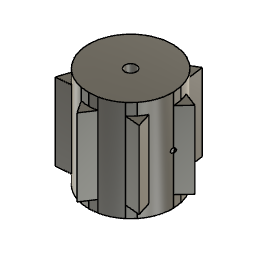
engranaje v5 (Autodesk Fusion 360 design; units mm, degrees)
Autodesk Fusion 360 part; units mm, degrees
sketch "Sketch1" plane through (0, 0, 0) normal (0, 0, 1) x (1, 0, 0)
  circle A0 centre (0, 0) radius 25
  line L0 (0, 25) -> (4.9749, 24.5)
  line L1 (0, 25) -> (-4.9749, 24.5)
  line L2 (0, -25) -> (0, -32)
  line L3 (0, -25) -> (-4.9749, -24.5)
  line L4 (0, -25) -> (0, -32)
  line L5 (0, -32) -> (-4.9749, -24.5)
  line L6 (0, -25) -> (4.9749, -24.5)
  line L7 (0, -32) -> (4.9749, -24.5)
  line L8 (25.0186, -19.9517) -> (16.053, -19.1651)
  line L9 (19.5458, -15.5872) -> (25.0186, -19.9517)
  line L10 (19.5458, -15.5872) -> (16.053, -19.1651)
  circle A1 centre (0, 0) radius 25
  line L11 (25.0186, -19.9517) -> (22.2567, -11.3859)
  line L12 (31.1977, 7.1207) -> (24.9928, 0.6016)
  line L13 (24.3732, 5.563) -> (31.1977, 7.1207)
  line L14 (24.3732, 5.563) -> (24.9928, 0.6016)
  circle A2 centre (0, 0) radius 25
  line L15 (31.1977, 7.1207) -> (22.7787, 10.302)
  line L16 (13.8843, 28.831) -> (15.1124, 19.9152)
  line L17 (10.8471, 22.5242) -> (13.8843, 28.831)
  line L18 (10.8471, 22.5242) -> (15.1124, 19.9152)
  circle A3 centre (0, 0) radius 25
  line L19 (13.8843, 28.831) -> (6.1479, 24.2323)
  line L20 (-13.8843, 28.831) -> (-6.1479, 24.2323)
  line L21 (-10.8471, 22.5242) -> (-13.8843, 28.831)
  line L22 (-10.8471, 22.5242) -> (-6.1479, 24.2323)
  circle A4 centre (0, 0) radius 25
  line L23 (-13.8843, 28.831) -> (-15.1124, 19.9152)
  line L24 (-31.1977, 7.1207) -> (-22.7787, 10.302)
  line L25 (-24.3732, 5.563) -> (-31.1977, 7.1207)
  line L26 (-24.3732, 5.563) -> (-22.7787, 10.302)
  circle A5 centre (0, 0) radius 25
  line L27 (-31.1977, 7.1207) -> (-24.9928, 0.6016)
  line L28 (-25.0186, -19.9517) -> (-22.2567, -11.3859)
  line L29 (-19.5458, -15.5872) -> (-25.0186, -19.9517)
  line L30 (-19.5458, -15.5872) -> (-22.2567, -11.3859)
  circle A6 centre (0, 0) radius 25
  line L31 (-25.0186, -19.9517) -> (-16.053, -19.1651)
  dimension "d1" = 50
  dimension "d2" = 5
  dimension "d3" = 7
  dimension "d4" = 5
  dimension "d5" = 5
  dimension "d7" = 360
  constraint coincident A0.centre A1.centre
  constraint coincident A0 L0.start
  constraint coincident A0 L0.end
  constraint coincident A0 L1.end
  constraint coincident A0 L2.start
  constraint vertical L2
  constraint coincident A0 L3.end
  constraint coincident A0 L6.end
  measures "d1" diameter of A0
  measures "d2" distance of L0.start L0.end
  measures "d3" distance of L2.start L2.end
  measures "d4" distance of L2.start L3.end
  measures "d5" distance of L2.start L6.end
extrude "Extrude1" add sketch "Sketch1" along normal blind 60 contours A0 L0 L1 L3 L6 L10 A1 L14 A2 L18 A3 L22 A4 L26 A5 L30 A6 | A0 A1 L12 L13 A2 A3 A4 A5 A6 | A0 L9 A1 L11 A2 A3 A4 A5 A6 | A0 A1 L13 A2 L15 A3 A4 A5 A6 | A0 L8 L9 A1 A2 A3 A4 A5 A6 | A0 A1 A2 L16 L17 A3 A4 A5 A6 | A0 L2 L4 L7 A1 A2 A3 A4 A5 A6 | A0 A1 A2 L17 A3 L19 A4 A5 A6 | A0 L2 L4 L5 A1 A2 A3 A4 A5 A6 | A0 A1 A2 A3 A4 A5 L29 A6 L31 | A0 A1 A2 A3 A4 A5 L28 L29 A6 | A0 A1 A2 A3 L20 L21 A4 A5 A6 | A0 A1 A2 A3 A4 L25 A5 L27 A6 | A0 A1 A2 A3 L21 A4 L23 A5 A6 | A0 A1 A2 A3 A4 L24 L25 A5 A6
sketch "Sketch2" plane through (0, 0, 60) normal (0, 0, 1) x (-1, 0, 0)
  arc A0 (6.1479, -24.2323) -> (10.8471, -22.5242) centre (0, 0) ccw
  line L0 (6.1479, -24.2323) -> (13.8843, -28.831)
  line L1 (13.8843, -28.831) -> (15.1124, -19.9152)
  arc A1 (15.1124, -19.9152) -> (22.7787, -10.302) centre (0, 0) ccw
  line L2 (22.7787, -10.302) -> (24.3732, -5.563)
  arc A2 (22.7787, -10.302) -> (24.3732, -5.563) centre (0, 0) ccw
  line L3 (22.7787, -10.302) -> (31.1977, -7.1207)
  line L4 (31.1977, -7.1207) -> (24.9928, -0.6016)
  arc A3 (24.9928, -0.6016) -> (22.2567, 11.3859) centre (0, 0) ccw
  line L5 (22.2567, 11.3859) -> (19.5458, 15.5872)
  arc A4 (22.2567, 11.3859) -> (19.5458, 15.5872) centre (0, 0) ccw
  line L6 (22.2567, 11.3859) -> (25.0186, 19.9517)
  line L7 (25.0186, 19.9517) -> (16.053, 19.1651)
  arc A5 (16.053, 19.1651) -> (4.9749, 24.5) centre (0, 0) ccw
  line L8 (4.9749, 24.5) -> (0, 25)
  line L9 (0, 25) -> (-4.9749, 24.5)
  arc A6 (-4.9749, 24.5) -> (-16.053, 19.1651) centre (0, 0) ccw
  line L10 (-16.053, 19.1651) -> (-19.5458, 15.5872)
  arc A7 (-16.053, 19.1651) -> (-19.5458, 15.5872) centre (0, 0) ccw
  line L11 (-16.053, 19.1651) -> (-25.0186, 19.9517)
  line L12 (-25.0186, 19.9517) -> (-22.2567, 11.3859)
  arc A8 (-22.2567, 11.3859) -> (-24.9928, -0.6016) centre (0, 0) ccw
  line L13 (-24.9928, -0.6016) -> (-24.3732, -5.563)
  arc A9 (-24.9928, -0.6016) -> (-24.3732, -5.563) centre (0, 0) ccw
  line L14 (-24.9928, -0.6016) -> (-31.1977, -7.1207)
  line L15 (-31.1977, -7.1207) -> (-22.7787, -10.302)
  arc A10 (-22.7787, -10.302) -> (-15.1124, -19.9152) centre (0, 0) ccw
  line L16 (-15.1124, -19.9152) -> (-10.8471, -22.5242)
  arc A11 (-15.1124, -19.9152) -> (-10.8471, -22.5242) centre (0, 0) ccw
  line L17 (-15.1124, -19.9152) -> (-13.8843, -28.831)
  line L18 (-13.8843, -28.831) -> (-6.1479, -24.2323)
  arc A12 (-6.1479, -24.2323) -> (-4.9749, -24.5) centre (0, 0) ccw
  line L19 (-4.9749, -24.5) -> (0, -25)
  line L20 (0, -25) -> (4.9749, -24.5)
  arc A13 (4.9749, -24.5) -> (6.1479, -24.2323) centre (0, 0) ccw
  line L21 (6.1479, -24.2323) -> (10.8471, -22.5242)
  circle A14 centre (0, 0) radius 32
  circle A15 centre (0, 0) radius 25
  constraint concentric A0 A14
  constraint coincident L14.end A14
  constraint concentric A0 A15
  constraint coincident L13.end A15
extrude "Extrude2" cut sketch "Sketch2" against normal blind 7 contours A0 L0 L1 A15 | L0 L18 A12 A13 A14 A15 | L1 A1 L3 A14 A15 | L15 A10 L17 A14 A15 | A11 L17 L18 A15 | A2 L3 L4 A15 | L4 A3 L6 A14 A15 | L12 A8 L14 A14 A15 | A9 L14 L15 A15 | L7 A5 A6 L11 A14 A15 | A7 L11 L12 A15 | A4 L6 L7 A15
sketch "Sketch3" plane through (0, 0, 0) normal (0, 0, -1) x (1, 0, 0)
  arc A0 (-10.8471, -22.5242) -> (-6.1479, -24.2323) centre (0, 0) ccw
  line L0 (-10.8471, -22.5242) -> (-6.1479, -24.2323)
  arc A1 (-6.1479, -24.2323) -> (-4.9749, -24.5) centre (0, 0) ccw
  line L1 (-4.9749, -24.5) -> (0, -25)
  line L2 (0, -25) -> (4.9749, -24.5)
  arc A2 (4.9749, -24.5) -> (6.1479, -24.2323) centre (0, 0) ccw
  line L3 (6.1479, -24.2323) -> (13.8843, -28.831)
  line L4 (13.8843, -28.831) -> (15.1124, -19.9152)
  arc A3 (10.8471, -22.5242) -> (15.1124, -19.9152) centre (0, 0) ccw
  line L5 (10.8471, -22.5242) -> (15.1124, -19.9152)
  arc A4 (15.1124, -19.9152) -> (22.7787, -10.302) centre (0, 0) ccw
  line L6 (22.7787, -10.302) -> (31.1977, -7.1207)
  line L7 (31.1977, -7.1207) -> (24.9928, -0.6016)
  arc A5 (24.3732, -5.563) -> (24.9928, -0.6016) centre (0, 0) ccw
  line L8 (24.3732, -5.563) -> (24.9928, -0.6016)
  arc A6 (24.9928, -0.6016) -> (22.2567, 11.3859) centre (0, 0) ccw
  line L9 (22.2567, 11.3859) -> (25.0186, 19.9517)
  line L10 (25.0186, 19.9517) -> (16.053, 19.1651)
  arc A7 (19.5458, 15.5872) -> (16.053, 19.1651) centre (0, 0) ccw
  line L11 (19.5458, 15.5872) -> (16.053, 19.1651)
  arc A8 (16.053, 19.1651) -> (4.9749, 24.5) centre (0, 0) ccw
  line L12 (4.9749, 24.5) -> (0, 25)
  line L13 (0, 25) -> (-4.9749, 24.5)
  arc A9 (-4.9749, 24.5) -> (-16.053, 19.1651) centre (0, 0) ccw
  line L14 (-16.053, 19.1651) -> (-25.0186, 19.9517)
  line L15 (-25.0186, 19.9517) -> (-22.2567, 11.3859)
  arc A10 (-19.5458, 15.5872) -> (-22.2567, 11.3859) centre (0, 0) ccw
  line L16 (-19.5458, 15.5872) -> (-22.2567, 11.3859)
  arc A11 (-22.2567, 11.3859) -> (-24.9928, -0.6016) centre (0, 0) ccw
  line L17 (-24.9928, -0.6016) -> (-31.1977, -7.1207)
  line L18 (-31.1977, -7.1207) -> (-22.7787, -10.302)
  arc A12 (-24.3732, -5.563) -> (-22.7787, -10.302) centre (0, 0) ccw
  line L19 (-24.3732, -5.563) -> (-22.7787, -10.302)
  arc A13 (-22.7787, -10.302) -> (-15.1124, -19.9152) centre (0, 0) ccw
  line L20 (-15.1124, -19.9152) -> (-13.8843, -28.831)
  line L21 (-13.8843, -28.831) -> (-6.1479, -24.2323)
  circle A14 centre (0, 0) radius 25
  circle A15 centre (0, 0) radius 32
  constraint concentric A0 A14
  constraint concentric A0 A15
  constraint coincident L9.end A15
extrude "Extrude3" cut sketch "Sketch3" against normal blind 7 contours A0 L20 L21 A14 | A1 A2 L3 L21 A14 A15 | L18 A13 L20 A14 A15 | L17 L18 A12 A14 | L15 A11 L17 A14 A15 | L3 L4 A3 A14 | L4 A4 L6 A14 A15 | L10 A8 A9 L14 A14 A15 | L14 L15 A10 A14 | L6 L7 A5 A14 | L7 A6 L9 A14 A15 | L9 L10 A7 A14
sketch "Sketch4" plane through (0, 0, 60) normal (0, 0, 1) x (-1, 0, 0)
  arc A0 (-10.8471, -22.5242) -> (-4.9749, -24.5) centre (0, 0) ccw
  line L0 (-4.9749, -24.5) -> (0, -25)
  line L1 (0, -25) -> (4.9749, -24.5)
  arc A1 (4.9749, -24.5) -> (6.1479, -24.2323) centre (0, 0) ccw
  line L2 (6.1479, -24.2323) -> (10.8471, -22.5242)
  arc A2 (10.8471, -22.5242) -> (22.7787, -10.302) centre (0, 0) ccw
  line L3 (22.7787, -10.302) -> (24.3732, -5.563)
  arc A3 (24.3732, -5.563) -> (22.2567, 11.3859) centre (0, 0) ccw
  line L4 (22.2567, 11.3859) -> (19.5458, 15.5872)
  arc A4 (19.5458, 15.5872) -> (4.9749, 24.5) centre (0, 0) ccw
  line L5 (4.9749, 24.5) -> (0, 25)
  line L6 (0, 25) -> (-4.9749, 24.5)
  arc A5 (-4.9749, 24.5) -> (-16.053, 19.1651) centre (0, 0) ccw
  line L7 (-16.053, 19.1651) -> (-19.5458, 15.5872)
  arc A6 (-19.5458, 15.5872) -> (-24.9928, -0.6016) centre (0, 0) ccw
  line L8 (-24.9928, -0.6016) -> (-24.3732, -5.563)
  arc A7 (-24.3732, -5.563) -> (-15.1124, -19.9152) centre (0, 0) ccw
  line L9 (-15.1124, -19.9152) -> (-10.8471, -22.5242)
  circle A8 centre (0, 0) radius 3.5
  dimension "d14" = 7
  constraint coincident A0.centre A1.centre
  measures "d14" diameter of A8
extrude "Extrude4" cut sketch "Sketch4" against normal blind 120 contours A8
sketch "Sketch5" plane through (0, 0, 0) normal (0, 1, 0) x (1, 0, 0)
  circle A0 centre (0, -30) radius 1.5
  dimension "d17" = 3
  measures "d17" diameter of A0
extrude "Extrude5" cut sketch "Sketch5" along normal blind 110 and the other way blind 0
sketch "Sketch6" plane through (0, 0, 0) normal (1, 0, 0) x (0, 1, 0)
  circle A0 centre (0, 30) radius 1.5
  dimension "d22" = 3
  measures "d22" diameter of A0
extrude "Extrude6" cut sketch "Sketch6" along normal blind 110 and the other way blind 80
thread "Thread1" "ISO Metric profile 3.0 M3x0.5 6H" major diameter 3.086 minor diameter 2.529 pitch 0.5 angle 60 resizes the face on face at (10.6402, 0.4746, 31.4229)
thread "Thread2" "ISO Metric profile 3.0 M3x0.5 6H" major diameter 3.086 minor diameter 2.529 pitch 0.5 angle 60 resizes the face on face at (-17.8737, 0.7299, 28.6896)
